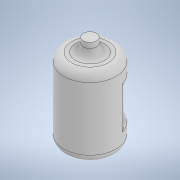
# Autodesk Inventor part: jug
Saved by Autodesk Inventor 2020.3 (Build 243373000, 373)
## iProperties
Created: 2021-03-04
Part Number: jug
Material: Generic
Document SubType Name: Modeling
Designer: con_c_000
Density: 1 g/cm^3
Appearance: Default
Author: con_c_000
Autodesk Inventor part; units mm, degrees
ref_plane "YZ Plane" through (0, 0, 0) normal (1, 0, 0) x (0, 1, 0)
ref_plane "XZ Plane" through (0, 0, 0) normal (0, 1, 0) x (-1, 0, 0)
ref_plane "XY Plane" through (0, 0, 0) normal (0, 0, 1) x (1, 0, 0)
sketch "Sketch1" plane through (0, 0, 0) normal (0, 1, 0) x (-1, 0, 0)
  circle A0 centre (0, 0) radius 127
  dimension "d0" = 254
  constraints: 1 centre point, 1 coincident
  measures "d0" diameter of A0
extrude "Extrusion1" add sketch "Sketch1" along normal blind 127
sketch "Sketch2" plane through (0, 127, 0) normal (0, 1, 0) x (1, 0, 0)
  circle A0 centre (0, 107.2156) radius 19.05
  circle A1 centre (0, 0) radius 127 projected
  line L0 (-97.6256, 53.539) -> (97.6256, 53.539)
  arc A2 (-122.032, 35.1737) -> (122.032, 35.1737) centre (0, 0) ccw
  arc A3 (-97.6256, 53.539) -> (-122.032, 35.1737) centre (-97.6256, 28.139) ccw
  arc A4 (122.032, 35.1737) -> (97.6256, 53.539) centre (97.6256, 28.139) ccw
  point P0 (-115.1633, 53.539)
  point P1 (115.1633, 53.539)
  point P2 (-122.032, 35.1737)
  point P3 (122.032, 35.1737)
  dimension "d3" = 38.1
  dimension "d4" = 25.4
  constraints: 10 point on circle, 4 centre point, 4 tangent, 2 end point, 2 equal radius, 2 point on line, 1 coincident, 1 horizontal
  measures "d3" diameter of A0
  measures "d4" radius of A3
extrude "Extrusion2" add sketch "Sketch2" along normal blind 127 contours A0 | A1 A3 L0 A4 picked at (-0.7658, -6.6337)
sketch "Sketch3" plane through (0, 254, 0) normal (0, 1, 0) x (1, 0, 0)
  circle A0 centre (0, 0) radius 127
  constraints: 1 centre point, 1 coincident
extrude "Extrusion3" add sketch "Sketch3" along normal blind 127
sketch "Sketch4" plane through (0, 381, 0) normal (0, 1, 0) x (1, 0, 0)
  circle A0 centre (0, 0) radius 31.75
  dimension "d9" = 63.5
  constraints: 1 centre point, 1 coincident
  measures "d9" diameter of A0
extrude "Extrusion4" add sketch "Sketch4" along normal blind 63.5
fillet "Fillet1" radius 38.1 1 edges at (-127, 381, 0)
fillet "Fillet2" radius 38.1 1 edges at (-31.75, 381, 0)
fillet "Fillet3" radius 38.1 1 edges at (127, 0, 0)
fillet "Fillet4" radius 38.1 2 edges at (0, 127, -127) (0, 254, -127)
body "Solid1"
